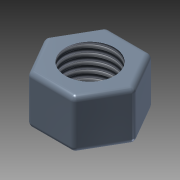
# Autodesk Inventor part: 集肉斗固定螺帽
Saved by Autodesk Inventor 2015 (Build 190159000, 159)
## iProperties
Created: 2017-05-22
Part Number: 集肉斗固定螺帽
Material: 常规
Document SubType Name: Modeling
Designer: Administrator
Density: 1 g/cm^3
Appearance: 钢蓝色
Author: Administrator
Autodesk Inventor part; units mm, degrees
ref_plane "YZ Plane" through (0, 0, 0) normal (1, 0, 0) x (0, 1, 0)
ref_plane "XZ Plane" through (0, 0, 0) normal (0, 1, 0) x (-1, 0, 0)
ref_plane "XY Plane" through (0, 0, 0) normal (0, 0, 1) x (1, 0, 0)
sketch "草图1" plane through (0, 0, 0) normal (0, 0, 1) x (1, 0, 0)
  line L0 (4.6188, -8) -> (-4.6188, -8)
  line L1 (-4.6188, -8) -> (-9.2376, 0)
  line L2 (-9.2376, 0) -> (-4.6188, 8)
  line L3 (-4.6188, 8) -> (4.6188, 8)
  line L4 (4.6188, 8) -> (9.2376, 0)
  line L5 (9.2376, 0) -> (4.6188, -8)
  line L6 (0, 0) -> (0, 8)
  circle A0 centre (0, 0) radius 5
  dimension "d0" = 16
  dimension "d1" = 10
  constraints: 14 end point, 2 coincident, 1 centre point, 1 midpoint, 1 vertical, 13 other
  measures "d0" distance between parallel lines of L0 L3
  measures "d1" diameter of A0
extrude "拉伸1" add sketch "草图1" along normal blind 10
thread "螺纹1" size "M10x1.5" class "6H" standard "ANSI Metric M Profile" full length
fillet "圆角1" radius 1 20 edges at (2.3094, 8, 10) (-2.3094, 8, 10) (-6.9282, 4, 10) (-6.9282, -4, 10) (0, -8, 10) (6.9282, -4, 10) (6.9282, 4, 10) (9.2376, 0, 5) (4.6188, 8, 5) (-4.6188, 8, 5) (-9.2376, 0, 5) (-4.6188, -8, 5) (4.6188, -8, 5) (6.9282, -4, 0) (6.9282, 4, 0) (2.3094, 8, 0) (-2.3094, 8, 0) (-6.9282, 4, 0) (-6.9282, -4, 0) (0, -8, 0)
